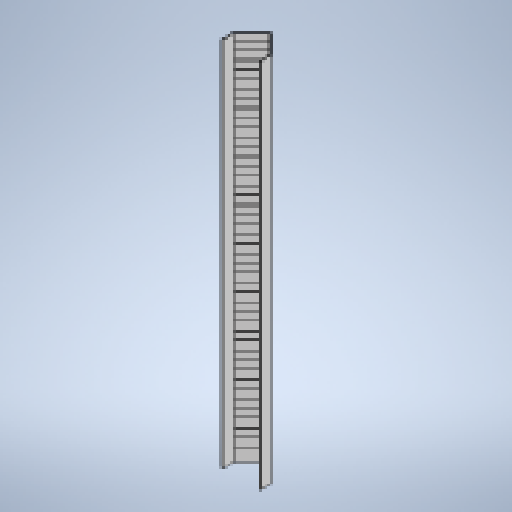
# Autodesk Inventor part: DSB-512 roof 2
Saved by Autodesk Inventor 2025.3 (Build 293356030, 356C)
## iProperties
Created: 2024-07-24
Part Number: DSB-512 roof 2
Material: Stainless Steel
Document SubType Name: Sheet Metal
Designer: admin
Density: 8 g/cm^3
Flat Pattern Width: 6.33321 cm
Flat Pattern Length: 31 cm
Flat Pattern Area: 196.33 cm^2
Sheet Metal Rule: Default
Sheet Metal Width: 63,332 mm
Sheet Metal Length: 310,000 mm
Sheet Metal Area: 19632,963 mm^2
Appearance: Default
Author: admin
Autodesk Inventor part; units mm, degrees
note: some values were not read from the file. Chosen so that the rebuilt part matches the saved one: flange form of "Plate1".
ref_plane "YZ Plane" through (0, 0, 0) normal (1, 0, 0) x (0, 1, 0)
ref_plane "XZ Plane" through (0, 0, 0) normal (0, 1, 0) x (-1, 0, 0)
ref_plane "XY Plane" through (0, 0, 0) normal (0, 0, 1) x (1, 0, 0)
sketch "Sketch3" plane through (0, 0, 0) normal (0, 0, 1) x (1, 0, 0)
  line L0 (-16, -10) -> (-16, -0.414214)
  line L1 (-16, 0) -> (-15.707107, 0.292893) construction
  line L2 (0, 16) -> (0.707107, 15.292893) construction
  line L3 (16, 0) -> (16, -0.414214) construction
  line L4 (0, 16) -> (0, 0) construction
  arc A0 (0.707107, 15.292893) -> (-0.707107, 15.292893) centre (0, 14.585786) ccw
  arc A1 (-15.707107, 0.292893) -> (-16, -0.414214) centre (-15, -0.414214) ccw
  arc A2 (16, -0.414214) -> (15.707107, 0.292893) centre (15, -0.414214) ccw
  line L5 (15.707107, 0.292893) -> (16, 0) construction
  line L6 (16, -0.414214) -> (16, -10)
  line L7 (-15.707107, 0.292893) -> (-0.707107, 15.292893)
  line L8 (-16, -0.414214) -> (-16, 0) construction
  line L9 (0.707107, 15.292893) -> (15.707107, 0.292893)
  line L10 (-0.707107, 15.292893) -> (0, 16) construction
  dimension "d15" = 10
  dimension "d18" = 1
  dimension "d19" = 1
  dimension "d20" = 1
  dimension "d32" = 32
  dimension "d33" = 90
  measures "d15" distance of L3.start L6.end
  measures "d18" radius of A0
  measures "d19" radius of A1
  measures "d20" radius of A2
  measures "d32" distance between parallel lines of L6 L0
  measures "d33" angle of L9 L7
contour flange "Contour Flange1" sketch "Sketch3" thickness 0.8 bend radius 0.8 width 310 along (0, 0, -1) mid plane no both sides no wall seen from (-16, -5.207107, 0) lies toward (1, 0, 0) curves L0 A1 L7 A0 L9 A2 L6
bend "Bend1"
corner "Corner1"
sketch "Sketch5" plane through (15.707107, 0.292893, 0) normal (0.7071068, 0.7071068, 0) x (-0.7071068, 0.7071068, 0)
  line L0 (0, -310) -> (0, 0) construction
  line L1 (0, 0) -> (21.213203, 0) construction
  line L2 (21.213203, 0) -> (21.213203, -310) construction
  line L3 (21.213203, -310) -> (0, -310) construction
  line L4 (20.713203, -5.1) -> (0.713203, -5.1) construction
  line L5 (20.713203, -5) -> (0.713203, -5)
  line L6 (0.713203, -5.2) -> (20.713203, -5.2)
  arc A0 (20.713203, -5.2) -> (20.713203, -5) centre (20.713203, -5.1) ccw
  arc A1 (0.713203, -5) -> (0.713203, -5.2) centre (0.713203, -5.1) ccw
  line L7 (20.713203, -12.1) -> (0.713203, -12.1) construction
  line L8 (20.713203, -12) -> (0.713203, -12)
  line L9 (0.713203, -12.2) -> (20.713203, -12.2)
  arc A2 (20.713203, -12.2) -> (20.713203, -12) centre (20.713203, -12.1) ccw
  arc A3 (0.713203, -12) -> (0.713203, -12.2) centre (0.713203, -12.1) ccw
  line L10 (20.713203, -19.1) -> (0.713203, -19.1) construction
  line L11 (20.713203, -19) -> (0.713203, -19)
  line L12 (0.713203, -19.2) -> (20.713203, -19.2)
  arc A4 (20.713203, -19.2) -> (20.713203, -19) centre (20.713203, -19.1) ccw
  arc A5 (0.713203, -19) -> (0.713203, -19.2) centre (0.713203, -19.1) ccw
  line L13 (20.713203, -26.1) -> (0.713203, -26.1) construction
  line L14 (20.713203, -26) -> (0.713203, -26)
  line L15 (0.713203, -26.2) -> (20.713203, -26.2)
  arc A6 (20.713203, -26.2) -> (20.713203, -26) centre (20.713203, -26.1) ccw
  arc A7 (0.713203, -26) -> (0.713203, -26.2) centre (0.713203, -26.1) ccw
  line L16 (20.713203, -33.1) -> (0.713203, -33.1) construction
  line L17 (20.713203, -33) -> (0.713203, -33)
  line L18 (0.713203, -33.2) -> (20.713203, -33.2)
  arc A8 (20.713203, -33.2) -> (20.713203, -33) centre (20.713203, -33.1) ccw
  arc A9 (0.713203, -33) -> (0.713203, -33.2) centre (0.713203, -33.1) ccw
  line L19 (20.713203, -40.1) -> (0.713203, -40.1) construction
  line L20 (20.713203, -40) -> (0.713203, -40)
  line L21 (0.713203, -40.2) -> (20.713203, -40.2)
  arc A10 (20.713203, -40.2) -> (20.713203, -40) centre (20.713203, -40.1) ccw
  arc A11 (0.713203, -40) -> (0.713203, -40.2) centre (0.713203, -40.1) ccw
  line L22 (20.713203, -47.1) -> (0.713203, -47.1) construction
  line L23 (20.713203, -47) -> (0.713203, -47)
  line L24 (0.713203, -47.2) -> (20.713203, -47.2)
  arc A12 (20.713203, -47.2) -> (20.713203, -47) centre (20.713203, -47.1) ccw
  arc A13 (0.713203, -47) -> (0.713203, -47.2) centre (0.713203, -47.1) ccw
  line L25 (20.713203, -54.1) -> (0.713203, -54.1) construction
  line L26 (20.713203, -54) -> (0.713203, -54)
  line L27 (0.713203, -54.2) -> (20.713203, -54.2)
  arc A14 (20.713203, -54.2) -> (20.713203, -54) centre (20.713203, -54.1) ccw
  arc A15 (0.713203, -54) -> (0.713203, -54.2) centre (0.713203, -54.1) ccw
  line L28 (20.713203, -61.1) -> (0.713203, -61.1) construction
  line L29 (20.713203, -61) -> (0.713203, -61)
  line L30 (0.713203, -61.2) -> (20.713203, -61.2)
  arc A16 (20.713203, -61.2) -> (20.713203, -61) centre (20.713203, -61.1) ccw
  arc A17 (0.713203, -61) -> (0.713203, -61.2) centre (0.713203, -61.1) ccw
  line L31 (20.713203, -68.1) -> (0.713203, -68.1) construction
  line L32 (20.713203, -68) -> (0.713203, -68)
  line L33 (0.713203, -68.2) -> (20.713203, -68.2)
  arc A18 (20.713203, -68.2) -> (20.713203, -68) centre (20.713203, -68.1) ccw
  arc A19 (0.713203, -68) -> (0.713203, -68.2) centre (0.713203, -68.1) ccw
  line L34 (20.713203, -75.1) -> (0.713203, -75.1) construction
  line L35 (20.713203, -75) -> (0.713203, -75)
  line L36 (0.713203, -75.2) -> (20.713203, -75.2)
  arc A20 (20.713203, -75.2) -> (20.713203, -75) centre (20.713203, -75.1) ccw
  arc A21 (0.713203, -75) -> (0.713203, -75.2) centre (0.713203, -75.1) ccw
  line L37 (20.713203, -82.1) -> (0.713203, -82.1) construction
  line L38 (20.713203, -82) -> (0.713203, -82)
  line L39 (0.713203, -82.2) -> (20.713203, -82.2)
  arc A22 (20.713203, -82.2) -> (20.713203, -82) centre (20.713203, -82.1) ccw
  arc A23 (0.713203, -82) -> (0.713203, -82.2) centre (0.713203, -82.1) ccw
  line L40 (20.713203, -89.1) -> (0.713203, -89.1) construction
  line L41 (20.713203, -89) -> (0.713203, -89)
  line L42 (0.713203, -89.2) -> (20.713203, -89.2)
  arc A24 (20.713203, -89.2) -> (20.713203, -89) centre (20.713203, -89.1) ccw
  arc A25 (0.713203, -89) -> (0.713203, -89.2) centre (0.713203, -89.1) ccw
  line L43 (20.713203, -96.1) -> (0.713203, -96.1) construction
  line L44 (20.713203, -96) -> (0.713203, -96)
  line L45 (0.713203, -96.2) -> (20.713203, -96.2)
  arc A26 (20.713203, -96.2) -> (20.713203, -96) centre (20.713203, -96.1) ccw
  arc A27 (0.713203, -96) -> (0.713203, -96.2) centre (0.713203, -96.1) ccw
  line L46 (20.713203, -103.1) -> (0.713203, -103.1) construction
  line L47 (20.713203, -103) -> (0.713203, -103)
  line L48 (0.713203, -103.2) -> (20.713203, -103.2)
  arc A28 (20.713203, -103.2) -> (20.713203, -103) centre (20.713203, -103.1) ccw
  arc A29 (0.713203, -103) -> (0.713203, -103.2) centre (0.713203, -103.1) ccw
  line L49 (20.713203, -110.1) -> (0.713203, -110.1) construction
  line L50 (20.713203, -110) -> (0.713203, -110)
  line L51 (0.713203, -110.2) -> (20.713203, -110.2)
  arc A30 (20.713203, -110.2) -> (20.713203, -110) centre (20.713203, -110.1) ccw
  arc A31 (0.713203, -110) -> (0.713203, -110.2) centre (0.713203, -110.1) ccw
  line L52 (20.713203, -117.1) -> (0.713203, -117.1) construction
  line L53 (20.713203, -117) -> (0.713203, -117)
  line L54 (0.713203, -117.2) -> (20.713203, -117.2)
  arc A32 (20.713203, -117.2) -> (20.713203, -117) centre (20.713203, -117.1) ccw
  arc A33 (0.713203, -117) -> (0.713203, -117.2) centre (0.713203, -117.1) ccw
  line L55 (20.713203, -124.1) -> (0.713203, -124.1) construction
  line L56 (20.713203, -124) -> (0.713203, -124)
  line L57 (0.713203, -124.2) -> (20.713203, -124.2)
  arc A34 (20.713203, -124.2) -> (20.713203, -124) centre (20.713203, -124.1) ccw
  arc A35 (0.713203, -124) -> (0.713203, -124.2) centre (0.713203, -124.1) ccw
  line L58 (20.713203, -131.1) -> (0.713203, -131.1) construction
  line L59 (20.713203, -131) -> (0.713203, -131)
  line L60 (0.713203, -131.2) -> (20.713203, -131.2)
  arc A36 (20.713203, -131.2) -> (20.713203, -131) centre (20.713203, -131.1) ccw
  arc A37 (0.713203, -131) -> (0.713203, -131.2) centre (0.713203, -131.1) ccw
  line L61 (20.713203, -138.1) -> (0.713203, -138.1) construction
  line L62 (20.713203, -138) -> (0.713203, -138)
  line L63 (0.713203, -138.2) -> (20.713203, -138.2)
  arc A38 (20.713203, -138.2) -> (20.713203, -138) centre (20.713203, -138.1) ccw
  arc A39 (0.713203, -138) -> (0.713203, -138.2) centre (0.713203, -138.1) ccw
  line L64 (20.713203, -145.1) -> (0.713203, -145.1) construction
  line L65 (20.713203, -145) -> (0.713203, -145)
  line L66 (0.713203, -145.2) -> (20.713203, -145.2)
  arc A40 (20.713203, -145.2) -> (20.713203, -145) centre (20.713203, -145.1) ccw
  arc A41 (0.713203, -145) -> (0.713203, -145.2) centre (0.713203, -145.1) ccw
  line L67 (20.713203, -152.1) -> (0.713203, -152.1) construction
  line L68 (20.713203, -152) -> (0.713203, -152)
  line L69 (0.713203, -152.2) -> (20.713203, -152.2)
  arc A42 (20.713203, -152.2) -> (20.713203, -152) centre (20.713203, -152.1) ccw
  arc A43 (0.713203, -152) -> (0.713203, -152.2) centre (0.713203, -152.1) ccw
  line L70 (20.713203, -159.1) -> (0.713203, -159.1) construction
  line L71 (20.713203, -159) -> (0.713203, -159)
  line L72 (0.713203, -159.2) -> (20.713203, -159.2)
  arc A44 (20.713203, -159.2) -> (20.713203, -159) centre (20.713203, -159.1) ccw
  arc A45 (0.713203, -159) -> (0.713203, -159.2) centre (0.713203, -159.1) ccw
  line L73 (20.713203, -166.1) -> (0.713203, -166.1) construction
  line L74 (20.713203, -166) -> (0.713203, -166)
  line L75 (0.713203, -166.2) -> (20.713203, -166.2)
  arc A46 (20.713203, -166.2) -> (20.713203, -166) centre (20.713203, -166.1) ccw
  arc A47 (0.713203, -166) -> (0.713203, -166.2) centre (0.713203, -166.1) ccw
  line L76 (20.713203, -173.1) -> (0.713203, -173.1) construction
  line L77 (20.713203, -173) -> (0.713203, -173)
  line L78 (0.713203, -173.2) -> (20.713203, -173.2)
  arc A48 (20.713203, -173.2) -> (20.713203, -173) centre (20.713203, -173.1) ccw
  arc A49 (0.713203, -173) -> (0.713203, -173.2) centre (0.713203, -173.1) ccw
  line L79 (20.713203, -180.1) -> (0.713203, -180.1) construction
  line L80 (20.713203, -180) -> (0.713203, -180)
  line L81 (0.713203, -180.2) -> (20.713203, -180.2)
  arc A50 (20.713203, -180.2) -> (20.713203, -180) centre (20.713203, -180.1) ccw
  arc A51 (0.713203, -180) -> (0.713203, -180.2) centre (0.713203, -180.1) ccw
  line L82 (20.713203, -187.1) -> (0.713203, -187.1) construction
  line L83 (20.713203, -187) -> (0.713203, -187)
  line L84 (0.713203, -187.2) -> (20.713203, -187.2)
  arc A52 (20.713203, -187.2) -> (20.713203, -187) centre (20.713203, -187.1) ccw
  arc A53 (0.713203, -187) -> (0.713203, -187.2) centre (0.713203, -187.1) ccw
  line L85 (20.713203, -194.1) -> (0.713203, -194.1) construction
  line L86 (20.713203, -194) -> (0.713203, -194)
  line L87 (0.713203, -194.2) -> (20.713203, -194.2)
  arc A54 (20.713203, -194.2) -> (20.713203, -194) centre (20.713203, -194.1) ccw
  arc A55 (0.713203, -194) -> (0.713203, -194.2) centre (0.713203, -194.1) ccw
  line L88 (20.713203, -201.1) -> (0.713203, -201.1) construction
  line L89 (20.713203, -201) -> (0.713203, -201)
  line L90 (0.713203, -201.2) -> (20.713203, -201.2)
  arc A56 (20.713203, -201.2) -> (20.713203, -201) centre (20.713203, -201.1) ccw
  arc A57 (0.713203, -201) -> (0.713203, -201.2) centre (0.713203, -201.1) ccw
  line L91 (20.713203, -208.1) -> (0.713203, -208.1) construction
  line L92 (20.713203, -208) -> (0.713203, -208)
  line L93 (0.713203, -208.2) -> (20.713203, -208.2)
  arc A58 (20.713203, -208.2) -> (20.713203, -208) centre (20.713203, -208.1) ccw
  arc A59 (0.713203, -208) -> (0.713203, -208.2) centre (0.713203, -208.1) ccw
  line L94 (20.713203, -215.1) -> (0.713203, -215.1) construction
  line L95 (20.713203, -215) -> (0.713203, -215)
  line L96 (0.713203, -215.2) -> (20.713203, -215.2)
  arc A60 (20.713203, -215.2) -> (20.713203, -215) centre (20.713203, -215.1) ccw
  arc A61 (0.713203, -215) -> (0.713203, -215.2) centre (0.713203, -215.1) ccw
  line L97 (20.713203, -222.1) -> (0.713203, -222.1) construction
  line L98 (20.713203, -222) -> (0.713203, -222)
  line L99 (0.713203, -222.2) -> (20.713203, -222.2)
  arc A62 (20.713203, -222.2) -> (20.713203, -222) centre (20.713203, -222.1) ccw
  arc A63 (0.713203, -222) -> (0.713203, -222.2) centre (0.713203, -222.1) ccw
  line L100 (20.713203, -229.1) -> (0.713203, -229.1) construction
  line L101 (20.713203, -229) -> (0.713203, -229)
  line L102 (0.713203, -229.2) -> (20.713203, -229.2)
  arc A64 (20.713203, -229.2) -> (20.713203, -229) centre (20.713203, -229.1) ccw
  arc A65 (0.713203, -229) -> (0.713203, -229.2) centre (0.713203, -229.1) ccw
  line L103 (20.713203, -236.1) -> (0.713203, -236.1) construction
  line L104 (20.713203, -236) -> (0.713203, -236)
  line L105 (0.713203, -236.2) -> (20.713203, -236.2)
  arc A66 (20.713203, -236.2) -> (20.713203, -236) centre (20.713203, -236.1) ccw
  arc A67 (0.713203, -236) -> (0.713203, -236.2) centre (0.713203, -236.1) ccw
  line L106 (20.713203, -243.1) -> (0.713203, -243.1) construction
  line L107 (20.713203, -243) -> (0.713203, -243)
  line L108 (0.713203, -243.2) -> (20.713203, -243.2)
  arc A68 (20.713203, -243.2) -> (20.713203, -243) centre (20.713203, -243.1) ccw
  arc A69 (0.713203, -243) -> (0.713203, -243.2) centre (0.713203, -243.1) ccw
  line L109 (20.713203, -250.1) -> (0.713203, -250.1) construction
  line L110 (20.713203, -250) -> (0.713203, -250)
  line L111 (0.713203, -250.2) -> (20.713203, -250.2)
  arc A70 (20.713203, -250.2) -> (20.713203, -250) centre (20.713203, -250.1) ccw
  arc A71 (0.713203, -250) -> (0.713203, -250.2) centre (0.713203, -250.1) ccw
  line L112 (20.713203, -257.1) -> (0.713203, -257.1) construction
  line L113 (20.713203, -257) -> (0.713203, -257)
  line L114 (0.713203, -257.2) -> (20.713203, -257.2)
  arc A72 (20.713203, -257.2) -> (20.713203, -257) centre (20.713203, -257.1) ccw
  arc A73 (0.713203, -257) -> (0.713203, -257.2) centre (0.713203, -257.1) ccw
  line L115 (20.713203, -264.1) -> (0.713203, -264.1) construction
  line L116 (20.713203, -264) -> (0.713203, -264)
  line L117 (0.713203, -264.2) -> (20.713203, -264.2)
  arc A74 (20.713203, -264.2) -> (20.713203, -264) centre (20.713203, -264.1) ccw
  arc A75 (0.713203, -264) -> (0.713203, -264.2) centre (0.713203, -264.1) ccw
  line L118 (20.713203, -271.1) -> (0.713203, -271.1) construction
  line L119 (20.713203, -271) -> (0.713203, -271)
  line L120 (0.713203, -271.2) -> (20.713203, -271.2)
  arc A76 (20.713203, -271.2) -> (20.713203, -271) centre (20.713203, -271.1) ccw
  arc A77 (0.713203, -271) -> (0.713203, -271.2) centre (0.713203, -271.1) ccw
  line L121 (20.713203, -278.1) -> (0.713203, -278.1) construction
  line L122 (20.713203, -278) -> (0.713203, -278)
  line L123 (0.713203, -278.2) -> (20.713203, -278.2)
  arc A78 (20.713203, -278.2) -> (20.713203, -278) centre (20.713203, -278.1) ccw
  arc A79 (0.713203, -278) -> (0.713203, -278.2) centre (0.713203, -278.1) ccw
  line L124 (20.713203, -285.1) -> (0.713203, -285.1) construction
  line L125 (20.713203, -285) -> (0.713203, -285)
  line L126 (0.713203, -285.2) -> (20.713203, -285.2)
  arc A80 (20.713203, -285.2) -> (20.713203, -285) centre (20.713203, -285.1) ccw
  arc A81 (0.713203, -285) -> (0.713203, -285.2) centre (0.713203, -285.1) ccw
  line L127 (20.713203, -292.1) -> (0.713203, -292.1) construction
  line L128 (20.713203, -292) -> (0.713203, -292)
  line L129 (0.713203, -292.2) -> (20.713203, -292.2)
  arc A82 (20.713203, -292.2) -> (20.713203, -292) centre (20.713203, -292.1) ccw
  arc A83 (0.713203, -292) -> (0.713203, -292.2) centre (0.713203, -292.1) ccw
  line L130 (20.713203, -299.1) -> (0.713203, -299.1) construction
  line L131 (20.713203, -299) -> (0.713203, -299)
  line L132 (0.713203, -299.2) -> (20.713203, -299.2)
  arc A84 (20.713203, -299.2) -> (20.713203, -299) centre (20.713203, -299.1) ccw
  arc A85 (0.713203, -299) -> (0.713203, -299.2) centre (0.713203, -299.1) ccw
  line L133 (20.713203, -306.1) -> (0.713203, -306.1) construction
  line L134 (20.713203, -306) -> (0.713203, -306)
  line L135 (0.713203, -306.2) -> (20.713203, -306.2)
  arc A86 (20.713203, -306.2) -> (20.713203, -306) centre (20.713203, -306.1) ccw
  arc A87 (0.713203, -306) -> (0.713203, -306.2) centre (0.713203, -306.1) ccw
  point P0 (10.899495, 0)
  point P1 (10.713203, -5.1)
  point P2 (10.713203, -12.1)
  point P3 (10.713203, -19.1)
  point P4 (10.713203, -26.1)
  point P5 (10.713203, -33.1)
  point P6 (10.713203, -40.1)
  point P7 (10.713203, -47.1)
  point P8 (10.713203, -54.1)
  point P9 (10.713203, -61.1)
  point P10 (10.713203, -68.1)
  point P11 (10.713203, -75.1)
  point P12 (10.713203, -82.1)
  point P13 (10.713203, -89.1)
  point P14 (10.713203, -96.1)
  point P15 (10.713203, -103.1)
  point P16 (10.713203, -110.1)
  point P17 (10.713203, -117.1)
  point P18 (10.713203, -124.1)
  point P19 (10.713203, -131.1)
  point P20 (10.713203, -138.1)
  point P21 (10.713203, -145.1)
  point P22 (10.713203, -152.1)
  point P23 (10.713203, -159.1)
  point P24 (10.713203, -166.1)
  point P25 (10.713203, -173.1)
  point P26 (10.713203, -180.1)
  point P27 (10.713203, -187.1)
  point P28 (10.713203, -194.1)
  point P29 (10.713203, -201.1)
  point P30 (10.713203, -208.1)
  point P31 (10.713203, -215.1)
  point P32 (10.713203, -222.1)
  point P33 (10.713203, -229.1)
  point P34 (10.713203, -236.1)
  point P35 (10.713203, -243.1)
  point P36 (10.713203, -250.1)
  point P37 (10.713203, -257.1)
  point P38 (10.713203, -264.1)
  point P39 (10.713203, -271.1)
  point P40 (10.713203, -278.1)
  point P41 (10.713203, -285.1)
  point P42 (10.713203, -292.1)
  point P43 (10.713203, -299.1)
  point P44 (10.713203, -306.1)
  dimension "d111" = 0.2
  dimension "d112" = 20
  dimension "d114" = 0.5
  dimension "d116" = 7
  dimension "d97" = 5
  constraints: 354 end point, 176 point on circle, 88 centre point, 4 tangent, 2 parallel, 1 midpoint, 1 perpendicular, 1 vertical, 516 other
  measures "d111" diameter of A1
  measures "d112" distance of L4.start L4.end
  measures "d114" distance from line of L4.start L2
  measures "d116" distance of L5.start L8.start
  measures "d97" distance between parallel lines of L5 L1
extrude "Cut3" cut sketch "Sketch5" against normal blind 0.8 contours A0 L6 A1 L5 | A2 L9 A3 L8 | A4 L12 A5 L11 | A6 L15 A7 L14 | A8 L18 A9 L17 | A10 L21 A11 L20 | A12 L24 A13 L23 | A14 L27 A15 L26 | A16 L30 A17 L29 | A18 L33 A19 L32 | A20 L36 A21 L35 | A22 L39 A23 L38 | A24 L42 A25 L41 | A26 L45 A27 L44 | A28 L48 A29 L47 | A30 L51 A31 L50 | A32 L54 A33 L53 | A34 L57 A35 L56 | A36 L60 A37 L59 | A38 L63 A39 L62 | A40 L66 A41 L65 | A42 L69 A43 L68 | A44 L72 A45 L71 | A46 L75 A47 L74 | A48 L78 A49 L77 | A50 L81 A51 L80 | A52 L84 A53 L83 | A54 L87 A55 L86 | A56 L90 A57 L89 | A58 L93 A59 L92 | A60 L96 A61 L95 | A62 L99 A63 L98 | A64 L102 A65 L101 | A66 L105 A67 L104 | A68 L108 A69 L107 | A70 L111 A71 L110 | A72 L114 A73 L113 | A74 L117 A75 L116 | A76 L120 A77 L119 | A78 L123 A79 L122 | A80 L126 A81 L125 | A82 L129 A83 L128 | A84 L132 A85 L131
mirror "Mirror2" about plane through (0, 0, 0) normal (1, 0, 0) of "Cut3"
equation "\"d21\" = Thickness"
equation "\"d22\" = BendReliefWidth"
equation "\"d23\" = BendReliefDepth"
equation "\"d24\" = MinimumRemnant"
equation "\"d25\" = TransitionRadius"
equation "\"d27\" = BendRadius"
equation "\"d29\" = CornerReliefSize"
equation "\"d30\" = GapSize"
equation "\"d31\" = JacobiRadiusSize"
equation "\"BendRadius\" = Thickness"
equation "\"BendReliefWidth\" = Thickness"
equation "\"BendReliefDepth\" = 0.5 * Thickness"
equation "\"CornerReliefSize\" = 4 * Thickness"
equation "\"MinimumRemnant\" = 2 * Thickness"
equation "\"TransitionRadius\" = BendRadius"
equation "\"JacobiRadiusSize\" = BendRadius"
equation "\"GapSize\" = Thickness"
equation "\"grat_thick\" = 0.2"
equation "\"grat_indet_X\" = 5"
equation "\"grat_indet_Y\" = 0.5"
equation "\"grat_number\" = 43.571429"
equation "\"grat_step\" = 7"
equation "\"BEAM_2_lenth\" = 335"
equation "\"BEAM_2_angle\" = 6deg"
equation "\"Thickness\" = 0.8"
body "Solid2"
